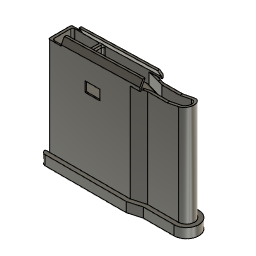
desert_tech_srs_magazine (Autodesk Fusion 360 design; units mm, degrees)
Autodesk Fusion 360 part; units mm, degrees
sketch "bottom_footprint" plane through (0, 0, 0) normal (0, 0, 1) x (1, 0, 0)
  line L0 (1.5, 0) -> (63.5, 0)
  line L1 (104.5, -3.8188) -> (104.5, 21.8188) construction
  line L2 (63.5, 18) -> (1.5, 18)
  line L3 (0, 16.25) -> (0, 1.5)
  line L4 (63.5, 18) -> (74, 15)
  line L5 (74, 15) -> (98, 15)
  line L6 (0, 9) -> (104.5, 9) construction
  arc A0 (104, 9) -> (98, 15) centre (98, 9) ccw
  line L7 (63.5, 0) -> (74, 3)
  line L8 (74, 3) -> (98, 3)
  arc A1 (98, 3) -> (104, 9) centre (98, 9) ccw
  line L9 (23.5, 15.5) -> (23.5, 10.6624)
  line L10 (25.5, 11.5003) -> (25.5, 15.5)
  line L11 (23.5, 2.5) -> (23.5, 7.3376)
  line L12 (25.5, 6.4997) -> (25.5, 2.5)
  arc A2 (100.0824, 12.4152) -> (98, 13) centre (98, 9) ccw
  line L13 (75.0019, 13) -> (98, 13)
  line L14 (61.0019, 17) -> (75.0019, 13)
  line L15 (2, 15.5) -> (2, 2.5)
  line L16 (61.014, 1) -> (75.014, 5)
  line L17 (75.014, 5) -> (98, 5)
  arc A3 (98, 5) -> (100.0824, 12.4152) centre (98, 9) ccw
  line L18 (61.0019, 17) -> (27, 17)
  line L19 (22, 17) -> (3.5, 17)
  line L20 (3.5, 1) -> (22, 1)
  line L21 (27, 1) -> (61.014, 1)
  line L22 (0, 1.5) -> (0, 0)
  line L23 (0, 0) -> (1.5, 0)
  line L24 (0, 16.25) -> (0, 18)
  line L25 (0, 18) -> (1.5, 18)
  line L26 (23.5, 10.6624) -> (23.5, 7.3376)
  line L27 (25.5, 11.5003) -> (25.5, 6.4997)
  arc A4 (27, 17) -> (25.5, 15.5) centre (27, 15.5) ccw
  arc A5 (25.5, 2.5) -> (27, 1) centre (27, 2.5) ccw
  arc A6 (23.5, 15.5) -> (22, 17) centre (22, 15.5) ccw
  arc A7 (22, 1) -> (23.5, 2.5) centre (22, 2.5) ccw
  arc A8 (3.5, 17) -> (2, 15.5) centre (3.5, 15.5) ccw
  arc A9 (2, 2.5) -> (3.5, 1) centre (3.5, 2.5) ccw
  point P0 (0, 18)
  dimension "d2" = 18
  dimension "d3" = 63.5
  dimension "d4" = 24
  dimension "d5" = 6.5
  dimension "d6" = 12
  dimension "d9" = 104.5
  dimension "d21" = 79
  dimension "d23" = 2
  dimension "d40" = 1
  dimension "d41" = 2
  dimension "d42" = 2
  dimension "d59" = 1.5
  dimension "d60" = 1.5
  dimension "d61" = 1.5
  dimension "d62" = 1.5
  dimension "d63" = 1.5
  dimension "d64" = 1.5
  dimension "d65" = 1
  constraint horizontal L0
  constraint vertical L1
  constraint horizontal L2
  constraint vertical L3
  constraint coincident L22.end L23.start
  constraint parallel L2 L5
  constraint midpoint L1 L6.end
  constraint coincident L6 A0.centre
  constraint tangent L5 A0
  constraint coincident L6 A0.start
  constraint symmetric L2.start L6 L0.end
  constraint symmetric L4.end L6 L7.end
  constraint symmetric L5.end L6 L8.end
  constraint symmetric L6 A0 A1
  constraint symmetric L6 A0.start A1.end
  constraint coincident L3 L6.start
  constraint coincident P0 L2
  constraint coincident P0 L3
  constraint coincident L22.end L3
  constraint coincident L22.end L0
  constraint symmetric L0 L2 L6
  constraint vertical L9
  constraint vertical L10
  constraint symmetric L6 L9.end L11.end
  constraint symmetric L6 L10.start L12.start
  constraint concentric A0 A2
  constraint parallel L5 L13
  constraint parallel L4 L14
  constraint parallel L2 L18
  constraint parallel L3 L15
  constraint parallel L0 L20
  constraint parallel L7 L16
  constraint parallel L8 L17
  constraint concentric A1 A3
  constraint tangent A2 A3
  constraint tangent A2 L13
  constraint tangent L17 A3
  constraint collinear L18 L19
  constraint collinear L20 L21
  constraint coincident P0 L24.end
  constraint parallel L12 L27
  constraint tangent L10 A4
  constraint tangent L18 A4
  constraint tangent L12 A5
  constraint tangent L21 A5
  constraint tangent L19 A6
  constraint tangent L9 A6
  constraint tangent L11 A7
  constraint tangent L20 A7
  constraint tangent L15 A8
  constraint tangent L19 A8
  constraint tangent L15 A9
  constraint tangent L20 A9
  constraint vertical L11
  measures "d2" distance of L22.end P0
  measures "d3" distance of L3 L2.start
  measures "d4" distance of L4.end L5.end
  measures "d5" distance of L1 L5.end
  measures "d6" diameter of A0
  measures "d9" distance of L1 L3
  measures "d21" distance of L1 L10
  measures "d23" distance of L9 L10
  measures "d40" distance of L2 L19
  measures "d41" distance of L5 L13
  measures "d42" distance of L3 L15
  measures "d59" radius of A4
  measures "d60" radius of A5
  measures "d61" radius of A6
  measures "d62" radius of A7
  measures "d63" radius of A8
  measures "d64" radius of A9
  measures "d65" distance of L0 L20
extrude "Extrude1" add sketch "bottom_footprint" along normal blind 80 makes body 1
sketch "latch_cut" plane through (0, 0, 0) normal (0, -1, 0) x (1, 0, 0)
  line L0 (0, 0) -> (63.5, 0)
  line L1 (63.5, 0) -> (63.5, 80)
  line L2 (63.5, 80) -> (0, 80)
  line L3 (28.5, 66) -> (40, 66)
  line L4 (40, 66) -> (40, 58.25)
  line L5 (40, 58.25) -> (28.5, 58.25)
  line L6 (28.5, 58.25) -> (28.5, 66)
  line L7 (0, 80) -> (0, 0)
  line L8 (0, 0) -> (0, 80)
  dimension "d25" = 7.75
  dimension "d26" = 11.5
  dimension "d28" = 14
  dimension "d36" = 28.5
  constraint horizontal L3
  constraint vertical L4
  constraint horizontal L5
  constraint vertical L6
  measures "d25" distance of L3 L5
  measures "d26" distance of L4 L6
  measures "d28" distance of L2 L3
  measures "d36" distance of L6 L8
extrude "Extrude2" cut sketch "latch_cut" against normal up to surface (1 mm away) contours L3 L4 L5 L6 bodies 1
sketch "feed_lip" plane through (0, 0, 0) normal (0, 1, 0) x (1, 0, 0)
  line L0 (0, -85) -> (70.8023, -87) construction
  line L1 (71, -80) -> (0, -80) construction
  line L2 (63.5, 0) -> (63.5, -80)
  line L3 (70.8023, -87) -> (71, -80)
  line L4 (63.5, -80) -> (74, -80)
  line L5 (0, -85) -> (0, -80) construction
  line L6 (10, -80) -> (10, -85.2825)
  line L7 (0, 0) -> (0, -80)
  line L8 (10, -85.2825) -> (70.8023, -87)
  line L9 (10, -80) -> (71, -80)
  point P0 (0, -80)
  dimension "d37" = 7
  dimension "d38" = 7.5
  dimension "d47" = 5
  dimension "d50" = 10
  constraint perpendicular L0 L3
  constraint coincident P0 L1.end
  constraint coincident L1.start L4
  constraint perpendicular L1 L5
  constraint coincident L1 L6.start
  constraint coincident L0 L6.end
  constraint perpendicular L1 L6
  measures "d37" distance of L0.end L1
  measures "d38" distance of L2.end L1.start
  measures "d47" distance of L1 L0.start
  measures "d50" distance of L6 L7
extrude "Extrude3" add sketch "feed_lip" along normal up to surface (18 mm away) bodies 1
sketch "feed_lip_cut" plane through (73.2014, 0, 2.0678) normal (0.999601, 0, 0.028236) x (0, 1, 0)
  line L0 (18, 77.9633) -> (18, 84.9661)
  line L1 (0, 84.9661) -> (0, 77.9633)
  line L2 (2.1429, 77.9633) -> (3.8531, 77.9633)
  line L3 (9, 88.91) -> (9, 61.5961) construction
  line L4 (1, 79.2975) -> (1, 77.9633)
  line L5 (0, 77.9633) -> (2.2125, 77.9633)
  line L6 (2.2125, 77.9633) -> (12.4801, 77.9633)
  line L7 (12.4801, 77.9633) -> (12.4801, 77.9631)
  line L8 (12.4801, 77.9631) -> (15.5375, 77.9631)
  line L9 (15.5375, 77.9631) -> (12.4801, 77.9632)
  line L10 (17.4429, 84.9661) -> (0, 84.9661)
  line L11 (0, 84.9661) -> (0, 77.9633)
  line L12 (1, 79.2975) -> (4.2, 84.9661)
  line L13 (0, 80.5773) -> (2.4775, 84.9661)
  line L14 (17, 79.2975) -> (13.8, 84.9661)
  line L15 (18, 80.5773) -> (15.5225, 84.9661)
  line L16 (17, 79.2975) -> (17, 77.9633)
  line L17 (18, 84.9661) -> (0, 84.9661)
  line L18 (0, 77.9633) -> (2.1429, 77.9633)
  line L19 (3.8531, 77.9633) -> (14.1434, 77.9633)
  line L20 (14.1434, 77.9633) -> (15.8571, 77.9633)
  line L21 (15.8571, 77.9633) -> (18, 77.9633)
  line L22 (18, 77.9633) -> (18, 84.9661)
  line L23 (18, 84.9661) -> (17.4429, 84.9661)
  dimension "d49" = 1.5
  dimension "d51" = 1
  dimension "d56" = 9.6
  constraint vertical L3
  constraint symmetric L0 L1 L3
  constraint coincident L10 L12.end
  constraint coincident L11 L13.start
  constraint coincident L10 L13.end
  constraint parallel L12 L13
  constraint parallel L1 L4
  constraint symmetric L3 L4.end L16.end
  constraint symmetric L3 L4.start L14.start
  constraint symmetric L3 L12.end L14.end
  constraint symmetric L3 L13.start L15.start
  constraint symmetric L3 L13.end L15.end
  constraint parallel L2 L6
  constraint parallel L1 L11
  constraint collinear L6 L19
  constraint horizontal L10
  constraint coincident L0.start L21.end
  constraint perpendicular L21 L22
  constraint coincident L15.start L22
  constraint collinear L10 L17
  constraint collinear L10 L23
  measures "d49" distance of L12 L13
  measures "d51" distance of L4 L11
  measures "d56" distance of L12.end L14.end
extrude "Extrude4" cut sketch "feed_lip_cut" along normal up to surface contours L0 L10 L15 L17 L22 L23 | L2 L4 L5 L6 L8 L9 L10 L12 L14 L16 L17 L18 L19 L20 L21 | L1 L10 L11 L13 L17 end surface through (10, 0, 80) normal (-1, 0, 0) offset 0 bodies 1
sketch "mgazine_plate_latch" plane through (0, 0, 0) normal (0, 0, -1) x (1, 0, 0)
  line L0 (61.0019, -17) -> (27, -17)
  line L1 (25.5, -15.5) -> (25.5, -2.5)
  line L2 (27, -1) -> (61.014, -1)
  line L3 (61.014, -1) -> (75.014, -5)
  line L4 (75.014, -5) -> (98, -5)
  arc A0 (98, -13) -> (98, -5) centre (98, -9) ccw
  line L5 (98, -13) -> (75.0019, -13)
  line L6 (75.0019, -13) -> (61.0019, -17)
  line L7 (2, -15.5) -> (2, -2.5)
  line L8 (23.5, -2.5) -> (23.5, -15.5)
  line L9 (0, 0) -> (0, -18)
  line L10 (0, -18) -> (63.5, -18)
  line L11 (63.5, -18) -> (74, -15)
  line L12 (74, -15) -> (98, -15)
  arc A1 (98, -15) -> (98, -3) centre (98, -9) ccw
  line L13 (98, -3) -> (74, -3)
  line L14 (74, -3) -> (63.5, 0)
  line L15 (63.5, 0) -> (0, 0)
  line L16 (0, -19.4407) -> (63.8085, -19.4407)
  line L17 (63.8085, -19.4407) -> (73.7522, -16.5997)
  line L18 (73.7522, -16.5997) -> (98, -16.5997)
  arc A2 (98, -16.5997) -> (98, -1.4003) centre (98, -9) ccw
  line L19 (98, -1.4003) -> (73.9484, -1.4003)
  line L20 (73.9484, -1.4003) -> (63.6749, 1.535)
  line L21 (63.6749, 1.535) -> (0, 1.535)
  line L22 (0, -18) -> (63.5, -18)
  line L23 (63.5, -18) -> (74, -15)
  line L24 (74, -15) -> (98, -15)
  arc A3 (98, -15) -> (98, -3) centre (98, -9) ccw
  line L25 (98, -3) -> (74, -3)
  line L26 (74, -3) -> (63.5, 0)
  line L27 (63.5, 0) -> (0, 0)
  line L28 (0, 0) -> (0, -18)
  line L29 (0, 0) -> (0, 1.535)
  line L30 (0, -18) -> (0, -19.4407)
  arc A4 (27, -1) -> (25.5, -2.5) centre (27, -2.5) ccw
  arc A5 (25.5, -15.5) -> (27, -17) centre (27, -15.5) ccw
  arc A6 (22, -17) -> (23.5, -15.5) centre (22, -15.5) ccw
  arc A7 (2, -15.5) -> (3.5, -17) centre (3.5, -15.5) ccw
  arc A8 (3.5, -1) -> (2, -2.5) centre (3.5, -2.5) ccw
  arc A9 (23.5, -2.5) -> (22, -1) centre (22, -2.5) ccw
  line L31 (22, -17) -> (3.5, -17)
  line L32 (3.5, -1) -> (22, -1)
  dimension "d53" = 0
  constraint coincident L9.start L15.end
  constraint perpendicular L21 L29
  constraint perpendicular L16 L30
  constraint parallel L10 L16
  constraint parallel L11 L17
  constraint parallel L12 L18
  constraint concentric A1 A2
  constraint parallel L13 L19
  constraint parallel L14 L20
  constraint parallel L15 L21
  constraint tangent A2 L19
  constraint tangent L18 A2
  measures "d53" distance of L10
extrude "Extrude5" add sketch "mgazine_plate_latch" against normal blind 2.8 contours L10 L11 L12 A1 L13 L14 L15 L16 L17 L18 A2 L19 L20 L21 L22 L23 L24 A3 L25 L26 L27 L29 L30 bodies 1
fillet "Fillet1" radius 1 4 edges at (0, 0, 41.4) (0, 18, 41.4) (0, -1.535, 1.4) (0, 19.4407, 1.4) on bodies 1
extrude "Extrude6" add 3 faces at (24.8585, 15.9663, 78.6966) (24.8333, 13.4867, 78.6958) (24.1667, 9.1534, 78.6771) along direction (-0.028236, 0, 0.999601) blind 2 on bodies 1 bodies 1
sketch "front_feed_ramp_helper" plane through (0, 3, 0) normal (0, -1, 0) x (1, 0, 0)
  line L0 (98, 2.8) -> (98, 80)
  line L1 (98, 80) -> (74, 80)
  line L2 (74, 80) -> (74, 2.8)
  line L3 (89, 80) -> (104, 83)
  line L4 (104, 83) -> (104, 80)
  line L5 (104, 80) -> (89, 80)
  line L6 (74, 2.8) -> (98, 2.8)
  dimension "d81" = 15
  dimension "d82" = 3
  constraint coincident L1 L3.start
  constraint perpendicular L1 L4
  constraint perpendicular L4 L5
  measures "d81" distance of L3.start L4.end
  measures "d82" distance of L3.end L4.end
extrude "Extrude7" add sketch "front_feed_ramp_helper" against normal up to surface (12 mm away) contours L1 L3 L4 L5 bodies 1
extrude "Extrude11" cut 3 faces at (102.8212, 13.8212, 80) (95, 10.3333, 80) (102.8212, 4.1788, 80) along direction (0, 0, -1) up to surface end surface through (89, 3, 80) normal (-0.196116, 0, 0.980581) offset 0 on bodies 1 bodies 1
ref_plane "WorkPlane2" through (0, 0, 70) normal (0, 0, 1) x (1, 0, 0)
sketch "follower_base" plane through (0, 0, 70) normal (0, 0, 1) x (1, 0, 0)
  arc A0 (1, 19.4407) -> (0, 18.4407) centre (1, 18.4407) ccw
  line L0 (1, 19.4407) -> (63.8085, 19.4407)
  line L1 (63.8085, 19.4407) -> (73.7522, 16.5997)
  line L2 (73.7522, 16.5997) -> (98, 16.5997)
  arc A1 (98, 1.4003) -> (98, 16.5997) centre (98, 9) ccw
  line L3 (98, 1.4003) -> (73.9484, 1.4003)
  line L4 (73.9484, 1.4003) -> (63.6749, -1.535)
  line L5 (63.6749, -1.535) -> (1, -1.535)
  arc A2 (0, -0.535) -> (1, -1.535) centre (1, -0.535) ccw
  line L6 (0, -0.535) -> (0, 18.4407)
  line L7 (25.5, 15.5) -> (25.5, 2.5)
  arc A3 (25.5, 2.5) -> (27, 1) centre (27, 2.5) ccw
  line L8 (27, 1) -> (61.014, 1)
  line L9 (61.014, 1) -> (75.014, 5)
  line L10 (75.014, 5) -> (98, 5)
  arc A4 (98, 5) -> (98, 13) centre (98, 9) ccw
  line L11 (98, 13) -> (75.0019, 13)
  line L12 (75.0019, 13) -> (61.0019, 17)
  line L13 (61.0019, 17) -> (27, 17)
  arc A5 (27, 17) -> (25.5, 15.5) centre (27, 15.5) ccw
  arc A6 (23.5, 15.5) -> (22, 17) centre (22, 15.5) ccw
  line L14 (22, 17) -> (3.5, 17)
  arc A7 (3.5, 17) -> (2, 15.5) centre (3.5, 15.5) ccw
  line L15 (2, 15.5) -> (2, 2.5)
  arc A8 (2, 2.5) -> (3.5, 1) centre (3.5, 2.5) ccw
  line L16 (3.5, 1) -> (22, 1)
  arc A9 (22, 1) -> (23.5, 2.5) centre (22, 2.5) ccw
  line L17 (23.5, 2.5) -> (23.5, 15.5)
  arc A10 (98, 5.8) -> (98, 12.2) centre (98, 9) ccw
  line L18 (98, 12.2) -> (74.8899, 12.2)
  line L19 (74.8899, 12.2) -> (60.8899, 16.2)
  line L20 (60.8899, 16.2) -> (27, 16.2)
  arc A11 (27, 16.2) -> (26.3, 15.5) centre (27, 15.5) ccw
  line L21 (26.3, 15.5) -> (26.3, 2.5)
  arc A12 (26.3, 2.5) -> (27, 1.8) centre (27, 2.5) ccw
  line L22 (27, 1.8) -> (60.902, 1.8)
  line L23 (60.902, 1.8) -> (74.902, 5.8)
  line L24 (74.902, 5.8) -> (98, 5.8)
  dimension "d85" = -0.8
extrude "Extrude12" add sketch "follower_base" along normal blind 2.5 separate body contours A10 L18 L19 L20 A11 L21 A12 L22 L23 L24 makes body 2
sketch "Sketch18" plane through (0, 0, 70) normal (0, 0, -1) x (1, 0, 0)
  line L0 (98, -5.8) -> (74.902, -5.8)
  line L1 (74.902, -5.8) -> (60.902, -1.8)
  line L2 (60.902, -1.8) -> (27, -1.8)
  arc A0 (27, -1.8) -> (26.3, -2.5) centre (27, -2.5) ccw
  line L3 (26.3, -2.5) -> (26.3, -15.5)
  arc A1 (26.3, -15.5) -> (27, -16.2) centre (27, -15.5) ccw
  line L4 (27, -16.2) -> (60.8899, -16.2)
  line L5 (60.8899, -16.2) -> (74.8899, -12.2)
  line L6 (74.8899, -12.2) -> (98, -12.2)
  arc A2 (98, -12.2) -> (98, -5.8) centre (98, -9) ccw
  line L7 (88, -12.2) -> (98, -12.2)
  arc A3 (98, -12.2) -> (98, -5.8) centre (98, -9) ccw
  line L8 (98, -5.8) -> (88, -5.8)
  line L9 (88, -5.8) -> (88, -12.2)
  line L10 (89, -11.2) -> (98, -11.2)
  arc A4 (98, -11.2) -> (98, -6.8) centre (98, -9) ccw
  line L11 (98, -6.8) -> (89, -6.8)
  line L12 (89, -6.8) -> (89, -11.2)
  dimension "d90" = 10
  dimension "d91" = -1
  constraint vertical L9
  constraint parallel L6 L7
  constraint concentric A2 A3
  constraint parallel L0 L8
  constraint tangent A3 L8
  measures "d90" distance of A2.centre L9
extrude "Extrude13" add sketch "Sketch18" along normal blind 10 contours L0 L6 A2 L7 A3 L8 L9 bodies 2
fillet "Fillet2" radius 0.5 1 faces at (49.5973, 6.6, 72.5) on bodies 2
sketch "Sketch20" plane through (0, 0, 0) normal (0, 0, 1) x (1, 0, 0)
  arc A0 (1, 19.4407) -> (0, 18.4407) centre (1, 18.4407) ccw
  line L0 (1, 19.4407) -> (63.8085, 19.4407)
  line L1 (63.8085, 19.4407) -> (73.7522, 16.5997)
  line L2 (73.7522, 16.5997) -> (98, 16.5997)
  arc A1 (98, 1.4003) -> (98, 16.5997) centre (98, 9) ccw
  line L3 (98, 1.4003) -> (73.9484, 1.4003)
  line L4 (73.9484, 1.4003) -> (63.6749, -1.535)
  line L5 (63.6749, -1.535) -> (1, -1.535)
  arc A2 (0, -0.535) -> (1, -1.535) centre (1, -0.535) ccw
  line L6 (0, -0.535) -> (0, 18.4407)
  arc A3 (23.5, 15.5) -> (22, 17) centre (22, 15.5) ccw
  line L7 (22, 17) -> (3.5, 17)
  arc A4 (3.5, 17) -> (2, 15.5) centre (3.5, 15.5) ccw
  line L8 (2, 15.5) -> (2, 2.5)
  arc A5 (2, 2.5) -> (3.5, 1) centre (3.5, 2.5) ccw
  line L9 (3.5, 1) -> (22, 1)
  arc A6 (22, 1) -> (23.5, 2.5) centre (22, 2.5) ccw
  line L10 (23.5, 2.5) -> (23.5, 15.5)
  line L11 (25.5, 15.5) -> (25.5, 2.5)
  arc A7 (25.5, 2.5) -> (27, 1) centre (27, 2.5) ccw
  line L12 (27, 1) -> (61.014, 1)
  line L13 (61.014, 1) -> (75.014, 5)
  line L14 (75.014, 5) -> (98, 5)
  arc A8 (98, 5) -> (98, 13) centre (98, 9) ccw
  line L15 (98, 13) -> (75.0019, 13)
  line L16 (75.0019, 13) -> (61.0019, 17)
  line L17 (61.0019, 17) -> (27, 17)
  arc A9 (27, 17) -> (25.5, 15.5) centre (27, 15.5) ccw
  line L18 (74.944, 5.5) -> (98, 5.5)
  arc A10 (98, 5.5) -> (98, 12.5) centre (98, 9) ccw
  line L19 (98, 12.5) -> (74.9319, 12.5)
  line L20 (74.9319, 12.5) -> (60.9319, 16.5)
  line L21 (60.9319, 16.5) -> (27, 16.5)
  arc A11 (27, 16.5) -> (26, 15.5) centre (27, 15.5) ccw
  line L22 (26, 15.5) -> (26, 2.5)
  arc A12 (26, 2.5) -> (27, 1.5) centre (27, 2.5) ccw
  line L23 (27, 1.5) -> (60.944, 1.5)
  line L24 (60.944, 1.5) -> (74.944, 5.5)
  dimension "d96" = -0.5
extrude "Extrude14" add sketch "Sketch20" along normal blind 2.5 separate body contours L18 A10 L19 L20 L21 A11 L22 A12 L23 L24 makes body 3
sketch "Sketch21" plane through (0, 0, 0) normal (0, 0, -1) x (1, 0, 0)
  line L0 (74.944, -5.5) -> (60.944, -1.5)
  line L1 (60.944, -1.5) -> (27, -1.5)
  arc A0 (27, -1.5) -> (26, -2.5) centre (27, -2.5) ccw
  line L2 (26, -2.5) -> (26, -15.5)
  arc A1 (26, -15.5) -> (27, -16.5) centre (27, -15.5) ccw
  line L3 (27, -16.5) -> (60.9319, -16.5)
  line L4 (60.9319, -16.5) -> (74.9319, -12.5)
  line L5 (74.9319, -12.5) -> (98, -12.5)
  arc A2 (98, -12.5) -> (98, -5.5) centre (98, -9) ccw
  line L6 (98, -5.5) -> (74.944, -5.5)
  circle A3 centre (48, -9) radius 5
  line L7 (28.44, -9) -> (77.44, -9) construction
  dimension "d99" = 10
  dimension "d100" = 22
  constraint horizontal L7
  constraint coincident A3.centre L7
  measures "d99" diameter of A3
  measures "d100" distance of L2 A3.centre
extrude "Extrude15" add sketch "Sketch21" along normal blind 3 contours A3 bodies 3
ref_plane "WorkPlane3" through (0, 0, 0) normal (0, 0, 1) x (1, 0, 0)
sketch "Sketch25" plane through (0, 0, 0) normal (0, 0, 1) x (1, 0, 0)
  arc A0 (1, 19.4407) -> (0, 18.4407) centre (1, 18.4407) ccw construction
  line L0 (1, 19.4407) -> (63.8085, 19.4407) construction
  line L1 (63.8085, 19.4407) -> (73.7522, 16.5997) construction
  line L2 (73.7522, 16.5997) -> (98, 16.5997) construction
  arc A1 (98, 1.4003) -> (98, 16.5997) centre (98, 9) ccw construction
  line L3 (98, 1.4003) -> (73.9484, 1.4003) construction
  line L4 (73.9484, 1.4003) -> (63.6749, -1.535) construction
  line L5 (63.6749, -1.535) -> (1, -1.535) construction
  arc A2 (0, -0.535) -> (1, -1.535) centre (1, -0.535) ccw construction
  line L6 (0, -0.535) -> (0, 18.4407) construction
  arc A3 (23.5, 15.5) -> (22, 17) centre (22, 15.5) ccw construction
  line L7 (22, 17) -> (3.5, 17) construction
  arc A4 (3.5, 17) -> (2, 15.5) centre (3.5, 15.5) ccw construction
  line L8 (2, 15.5) -> (2, 2.5) construction
  arc A5 (2, 2.5) -> (3.5, 1) centre (3.5, 2.5) ccw construction
  line L9 (3.5, 1) -> (22, 1) construction
  arc A6 (22, 1) -> (23.5, 2.5) centre (22, 2.5) ccw construction
  line L10 (23.5, 2.5) -> (23.5, 15.5) construction
  line L11 (25.5, 15.5) -> (25.5, 2.5) construction
  arc A7 (25.5, 2.5) -> (27, 1) centre (27, 2.5) ccw construction
  line L12 (27, 1) -> (61.014, 1) construction
  line L13 (61.014, 1) -> (75.014, 5) construction
  line L14 (75.014, 5) -> (98, 5) construction
  arc A8 (98, 5) -> (98, 13) centre (98, 9) ccw construction
  line L15 (98, 13) -> (75.0019, 13) construction
  line L16 (75.0019, 13) -> (61.0019, 17) construction
  line L17 (61.0019, 17) -> (27, 17) construction
  arc A9 (27, 17) -> (25.5, 15.5) centre (27, 15.5) ccw construction
  circle A10 centre (48, 9) radius 5 construction
  arc A11 (-2, -0.535) -> (1, -3.535) centre (1, -0.535) ccw
  line L18 (63.955, -3.535) -> (1, -3.535)
  line L19 (74.2285, -0.5997) -> (63.955, -3.535)
  line L20 (98, -0.5997) -> (74.2285, -0.5997)
  arc A12 (98, -0.5997) -> (98, 18.5997) centre (98, 9) ccw
  line L21 (74.0323, 18.5997) -> (98, 18.5997)
  line L22 (64.0886, 21.4407) -> (74.0323, 18.5997)
  line L23 (1, 21.4407) -> (64.0886, 21.4407)
  arc A13 (1, 21.4407) -> (-2, 18.4407) centre (1, 18.4407) ccw
  line L24 (-2, -0.535) -> (-2, 18.4407)
  circle A14 centre (48, 9) radius 5.5
  dimension "d108" = -2
  dimension "d109" = 0.5
  measures "d108" distance of A2
extrude "Extrude16" add sketch "Sketch25" against normal blind 3 separate body makes body 4
sketch "Sketch26" plane through (0, 0, 0) normal (0, 0, 1) x (-1, 0, 0)
  arc A0 (-98, 0.5997) -> (-98, -18.5997) centre (-98, -9) ccw
  line L0 (-98, -18.5997) -> (-74.0323, -18.5997)
  line L1 (-74.0323, -18.5997) -> (-64.0886, -21.4407)
  line L2 (-64.0886, -21.4407) -> (-1, -21.4407)
  arc A1 (-1, -21.4407) -> (2, -18.4407) centre (-1, -18.4407) ccw
  line L3 (2, -18.4407) -> (2, 0.535)
  arc A2 (2, 0.535) -> (-1, 3.535) centre (-1, 0.535) ccw
  line L4 (-1, 3.535) -> (-63.955, 3.535)
  line L5 (-63.955, 3.535) -> (-74.2285, 0.5997)
  line L6 (-74.2285, 0.5997) -> (-98, 0.5997)
  line L7 (-2, -17.4407) -> (-2, -0.465)
  line L8 (-2, -0.465) -> (-63.3948, -0.465)
  line L9 (-63.3948, -0.465) -> (-73.6683, -3.4003)
  line L10 (-73.6683, -3.4003) -> (-98, -3.4003)
  arc A3 (-98, -3.4003) -> (-98, -14.5997) centre (-98, -9) ccw
  line L11 (-98, -14.5997) -> (-73.4721, -14.5997)
  line L12 (-73.4721, -14.5997) -> (-63.5284, -17.4407)
  line L13 (-63.5284, -17.4407) -> (-2, -17.4407)
  line L14 (2, -18.4407) -> (2, 0.535)
  arc A4 (2, 0.535) -> (-1, 3.535) centre (-1, 0.535) ccw
  line L15 (-1, 3.535) -> (-63.955, 3.535)
  line L16 (-63.955, 3.535) -> (-74.2285, 0.5997)
  line L17 (-74.2285, 0.5997) -> (-98, 0.5997)
  arc A5 (-98, 0.5997) -> (-98, -18.5997) centre (-98, -9) ccw
  line L18 (-98, -18.5997) -> (-74.0323, -18.5997)
  line L19 (-74.0323, -18.5997) -> (-64.0886, -21.4407)
  line L20 (-64.0886, -21.4407) -> (-1, -21.4407)
  arc A6 (-1, -21.4407) -> (2, -18.4407) centre (-1, -18.4407) ccw
  circle A7 centre (-48, -9) radius 5.5
  dimension "d113" = -4
  dimension "d114" = 0
  measures "d114" distance of L3
extrude "Extrude17" add sketch "Sketch26" along normal blind 4.5 contours A0 L0 L1 L2 A1 L3 A2 L4 L5 L6 L14 A4 L15 L16 L17 A5 L18 L19 L20 A6 bodies 4
combine "Combine2" operation cut target body 4 tool bodies 1 keep tools
sketch "Sketch32" plane through (0, 0, 4.5) normal (0, 0, 1) x (-1, 0, 0)
  arc A0 (-1, -18) -> (0, -17) centre (-1, -17) ccw
  line L0 (-1, -18) -> (-63.5, -18)
  line L1 (-63.5, -18) -> (-74, -15)
  line L2 (-74, -15) -> (-98, -15)
  arc A1 (-98, -3) -> (-98, -15) centre (-98, -9) ccw
  line L3 (-98, -3) -> (-74, -3)
  line L4 (-74, -3) -> (-63.5, 0)
  line L5 (-63.5, 0) -> (-1, 0)
  arc A2 (0, -1) -> (-1, 0) centre (-1, -1) ccw
  line L6 (0, -1) -> (0, -17)
  arc A3 (-1, -21.4407) -> (2, -18.4407) centre (-1, -18.4407) ccw
  line L7 (2, -18.4407) -> (2, 0.535)
  arc A4 (2, 0.535) -> (-1, 3.535) centre (-1, 0.535) ccw
  line L8 (-1, 3.535) -> (-63.955, 3.535)
  line L9 (-63.955, 3.535) -> (-74.2285, 0.5997)
  line L10 (-74.2285, 0.5997) -> (-98, 0.5997)
  arc A5 (-98, 0.5997) -> (-98, -18.5997) centre (-98, -9) ccw
  line L11 (-98, -18.5997) -> (-74.0323, -18.5997)
  line L12 (-74.0323, -18.5997) -> (-64.0886, -21.4407)
  line L13 (-64.0886, -21.4407) -> (-1, -21.4407)
  line L14 (-1, -18) -> (2, -18)
  line L15 (2, -18) -> (2, 0)
  line L16 (2, 0) -> (-1, 0)
  line L17 (-1, 0) -> (-1, -18)
  constraint horizontal L14
  constraint vertical L15
  constraint horizontal L16
  constraint vertical L17
  constraint coincident L7 L15.end
  constraint coincident A0.start L0.start
  constraint collinear L5 L16
extrude "Extrude21" cut sketch "Sketch32" against normal up to surface (1.7 mm away) contours A0 A2 L6 L17 | A0 A2 L6 L7 L14 L15 L16 bodies 4
sketch "Sketch33" plane through (0, 0, 0) normal (0, 0, 1) x (-1, 0, 0)
  arc A0 (-1, -19.4407) -> (0, -18.4407) centre (-1, -18.4407) ccw
  line L0 (0, -18.4407) -> (0, 0.535)
  arc A1 (0, 0.535) -> (-1, 1.535) centre (-1, 0.535) ccw
  line L1 (-1, 1.535) -> (-63.6749, 1.535)
  line L2 (-63.6749, 1.535) -> (-73.9484, -1.4003)
  line L3 (-73.9484, -1.4003) -> (-98, -1.4003)
  arc A2 (-98, -1.4003) -> (-98, -16.5997) centre (-98, -9) ccw
  line L4 (-98, -16.5997) -> (-73.7522, -16.5997)
  line L5 (-73.7522, -16.5997) -> (-63.8085, -19.4407)
  line L6 (-63.8085, -19.4407) -> (-1, -19.4407)
  circle A3 centre (-48, -9) radius 5.5
  line L7 (-1, -19.4407) -> (2, -19.4407)
  line L8 (2, -19.4407) -> (2, 1.535)
  line L9 (2, 1.535) -> (-1, 1.535)
  line L10 (-1, 1.535) -> (-1, -19.4407)
  line L11 (2, 0) -> (2, -18)
  constraint horizontal L7
  constraint vertical L8
  constraint horizontal L9
  constraint vertical L10
  constraint coincident A0.start L6.end
  constraint coincident A1.end L9
  constraint collinear L8 L11
extrude "Extrude22" cut sketch "Sketch33" along normal up to surface (2.8 mm away) contours A0 L0 A1 L10 | A0 L0 A1 L7 L8 L9 L11 bodies 4
move_face "OffsetFaces1" offset -0.4 7 faces at (20.006, -1.535, 0.9333) (70.5239, 0.4219, 0.9333) (89.9828, 1.4003, 0.9333) (104.9271, 5.8744, 1.8667) (41.9295, 19.4407, 0.9333) (67.1231, 18.4937, 0.9333) (81.8348, 16.5997, 0.9333) on bodies 4
move_face "OffsetFaces2" offset -0.4 1 faces at (12.8333, 8.9686, 0) on bodies 4
move_face "OffsetFaces3" offset -0.3 7 faces at (67, 17, 3.3667) (90, 15, 3.9333) (41.6667, 18, 3.9333) (100.3306, 3.4711, 3.9333) (90, 3, 3.3667) (70.5, 2, 3.9333) (19.8333, 0, 3.9333) on bodies 4
named bodies: "magazine_body", "magazine_follower", "base_pad_latch", "magazine_base"
